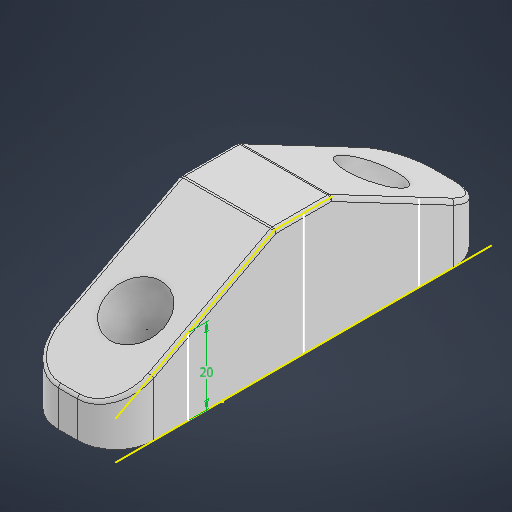
# Autodesk Inventor part: Bottom_End_Top
Saved by Autodesk Inventor 2026.2 (Build 302298000, 298)
## iProperties
Created: 2025-12-10
Part Number: Bottom_End_Top
Material: Generic
Document SubType Name: Modeling
Designer: Thoma
Density: 1 g/cm^3
Appearance: Default
Author: Thoma
Autodesk Inventor part; units mm, degrees
ref_plane "YZ Plane" through (0, 0, 0) normal (1, 0, 0) x (0, 1, 0)
ref_plane "XZ Plane" through (0, 0, 0) normal (0, 1, 0) x (-1, 0, 0)
ref_plane "XY Plane" through (0, 0, 0) normal (0, 0, 1) x (1, 0, 0)
sketch "Sketch1" plane through (0, 0, 0) normal (0, 1, 0) x (-1, 0, 0)
  line L0 (16.5841, 27.9312) -> (-8.4159, 27.9312)
  line L1 (-8.4159, 27.9312) -> (-8.4159, -70.7008)
  line L2 (-8.4159, -70.7008) -> (16.5841, -70.7008)
  line L3 (16.5841, -70.7008) -> (16.5841, 27.9312)
  line L4 (16.5841, -21.3848) -> (-8.4159, -21.3848)
  circle A0 centre (4.0841, -61.2943) radius 5
  line L5 (4.0841, -21.3848) -> (4.0841, -61.2943)
  line L6 (-8.4159, 27.9312) -> (16.5841, 27.9312)
  circle A1 centre (4.0841, 18.5247) radius 5
  point P0 (0, 0)
  dimension "d0" = 98.632
  dimension "d1" = 25
  dimension "d2" = 39.9095
  dimension "d3" = 10
  constraints: 14 end point, 3 midpoint, 2 centre point, 2 parallel, 1 horizontal, 1 perpendicular, 1 symmetric about line, 1 vertical, 1 other
  measures "d0" distance of L2.end L0.start
  measures "d1" distance of L1.end L2.end
  measures "d2" distance of L5.start L5.end
  measures "d3" diameter of A0
extrude "Extrusion1" add sketch "Sketch1" along normal blind 10
sketch "Sketch2" plane through (8.4159, 0, 27.9312) normal (1, 0, 0) x (0, 0, -1)
  line L0 (41.816, 10) -> (56.816, 10)
  line L1 (56.816, 10) -> (56.816, 32)
  line L2 (56.816, 32) -> (41.816, 32)
  line L3 (41.816, 32) -> (41.816, 10)
  line L4 (49.316, 10) -> (49.316, 0)
  line L5 (98.632, 0) -> (0, 0) projected
  line L6 (49.316, 0) -> (49.316, 10)
  point P0 (27.9312, 0)
  dimension "d6" = 22
  dimension "d7" = 15
  dimension "d8" = 0
  constraints: 12 end point, 4 midpoint, 2 parallel, 2 perpendicular, 1 horizontal, 1 vertical
  measures "d6" distance of L0.end L1.end
  measures "d7" distance of L1.end L2.end
  measures "d8" distance between parallel lines of L6 L4
extrude "Extrusion2" add sketch "Sketch2" against normal blind 25
sketch "Sketch12" plane through (8.4159, 0, 27.9312) normal (1, 0, 0) x (0, 0, -1)
  line L0 (41.816, 10) -> (41.816, 32) projected
  line L1 (0, 0) -> (0, 10) projected
  line L2 (41.816, 32) -> (0, 10)
  line L3 (0, 10) -> (41.816, 10)
  line L4 (41.816, 10) -> (41.816, 32)
  line L5 (41.816, 32) -> (56.816, 32) projected
  line L6 (56.816, 32) -> (56.816, 10) projected
  line L7 (56.816, 32) -> (56.816, 10)
  line L8 (98.632, 0) -> (98.632, 10) projected
  line L9 (56.816, 10) -> (98.632, 10)
  line L10 (98.632, 10) -> (56.816, 32)
  point P0 (27.9312, 0)
  constraints: 12 end point, 3 perpendicular, 1 vertical
extrude "Extrusion8" add sketch "Sketch12" against normal blind 25
sketch "Sketch13" plane through (8.4159, 0, 27.9312) normal (1, 0, 0) x (0, 0, -1)
  line L0 (41.816, 32) -> (0, 10) projected
  line L1 (19.0073, 20) -> (19.0073, 0)
  line L2 (98.632, 0) -> (0, 0) projected
  line L3 (56.816, 32) -> (41.816, 32) projected
  line L4 (49.316, 32) -> (49.316, 0)
  line L5 (79.6247, 20) -> (79.6247, 0)
  point P0 (27.9312, 0)
  dimension "d36" = 20
  constraints: 6 end point, 2 midpoint, 2 point on line, 2 symmetric about line, 1 vertical
  measures "d36" distance of L1.start L1.end
sketch "Sketch14" plane through (-16.5841, 32, -13.8848) normal (0, 0.8849917, 0.4656069) x (1, 0, 0)
  line L0 (25, 0) -> (25, -47.2502) projected
  line L1 (25, -27.1874) -> (0, -27.1874)
  circle A0 centre (12.5, -27.1874) radius 7.5
  point P0 (16.5841, -27.1874)
  dimension "d37" = 15
  constraints: 2 end point, 1 centre point, 1 horizontal, 1 midpoint, 1 point on line
  measures "d37" diameter of A0
extrude "Extrusion9" cut sketch "Sketch14" against normal blind 6.5
sketch "Sketch15" plane through (-16.5841, 10, -70.7008) normal (0, 0.8849917, -0.4656069) x (1, 0, 0)
  line L0 (25, 0) -> (25, -47.2502) projected
  line L1 (25, -21.4773) -> (0, -21.4773)
  line L2 (0, -47.2502) -> (0, 0) projected
  circle A0 centre (12.5, -21.4773) radius 7.5
  point P0 (16.5841, -57.9136)
  dimension "d41" = 15
  constraints: 2 end point, 2 point on line, 1 centre point, 1 horizontal, 1 midpoint
  measures "d41" diameter of A0
extrude "Extrusion10" cut sketch "Sketch15" against normal blind 6.5
fillet "Fillet5" radius 10 4 edges at (-16.5841, 5, 27.9312) (8.4159, 5, 27.9312) (-16.5841, 5, -70.7008) (8.4159, 5, -70.7008)
fillet "Fillet6" radius 1 14 edges at (5.4869, 11.541, -67.7719) (-4.0841, 10, -70.7008) (-13.6552, 11.541, -67.7719) (-16.5841, 23.6306, -44.7928) (-4.0841, 32, -28.8848) (8.4159, 23.6306, -44.7928) (5.4869, 11.541, 25.0023) (8.4159, 23.6306, 2.0232) (-4.0841, 32, -13.8848) (-16.5841, 23.6306, 2.0232) (-13.6552, 11.541, 25.0023) (-4.0841, 10, 27.9312) (-16.5841, 32, -21.3848) (8.4159, 32, -21.3848)
sketch "Sketch16" plane through (8.4159, 0, 17.9312) normal (1, 0, 0) x (0, 0, -1)
  line L0 (39.316, 33.3763) -> (39.316, 14.6237)
  line L1 (0, 0) -> (78.632, 0) projected
  line L2 (39.316, 14.6237) -> (39.316, 0)
  circle A0 centre (39.316, 24) radius 5
  circle A1 centre (39.316, 7.3119) radius 5
  point P0 (17.9312, 0)
  dimension "d47" = 10
  dimension "d48" = 10
  constraints: 4 end point, 3 midpoint, 2 centre point
  measures "d47" diameter of A0
  measures "d48" diameter of A1
extrude "Extrusion11" add sketch "Sketch16" against normal blind 10
fillet "Fillet7" radius 7.5 2 edges at (-11.5841, 13.5872, 7.1484) (-11.5841, 14.2458, -48.6662)
body "Solid1"
